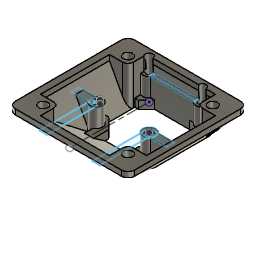
FanMod v4 (Autodesk Fusion 360 design; units mm, degrees)
Autodesk Fusion 360 part; units mm, degrees
note: some values were not read from the file. Chosen so that the rebuilt part matches the saved one: where a step ends; which bodies a step acts on; which sketch regions a step uses; which face or edge a step refers to.
sketch "2510Screws" plane through (0, 0, 0) normal (0, 0, 1) x (1, 0, 0)
  line L0 (12.5, -12.5) -> (-12.5, -12.5) construction
  line L1 (-12.5, -12.5) -> (-12.5, 12.5) construction
  line L2 (-12.5, 12.5) -> (12.5, 12.5) construction
  line L3 (12.5, 12.5) -> (12.5, -12.5) construction
  line L4 (12.5, -12.5) -> (-12.5, 12.5) construction
  line L5 (-12.5, -12.5) -> (12.5, 12.5) construction
  line L6 (10, -10) -> (-10, -10) construction
  line L7 (-10, -10) -> (-10, 10) construction
  line L8 (-10, 10) -> (10, 10) construction
  line L9 (10, 10) -> (10, -10) construction
  line L10 (10, -10) -> (-10, 10) construction
  line L11 (-10, -10) -> (10, 10) construction
  circle A0 centre (-10, 10) radius 1.4
  circle A1 centre (-10, -10) radius 1.4
  circle A2 centre (10, -10) radius 1.4
  circle A3 centre (10, 10) radius 1.4
  circle A4 centre (-10, 10) radius 2.4
  circle A5 centre (10, 10) radius 2.4
  circle A6 centre (-10, -10) radius 2.4
  circle A7 centre (10, -10) radius 2.4
  dimension "d1" = 25
  dimension "d2" = 25
  dimension "d3" = 20
  dimension "d4" = 20
  dimension "d5" = 2.8
  dimension "d6" = 2.8
  dimension "d7" = 2.8
  dimension "d8" = 2.8
  dimension "d9" = 4.8
  dimension "d10" = 4.8
  dimension "d11" = 4.8
  dimension "d12" = 4.8
  constraint horizontal L0
  constraint perpendicular L0 L1
  constraint parallel L0 L2
  constraint parallel L1 L3
  constraint coincident L4 origin
  constraint coincident L5 origin
  constraint horizontal L6
  constraint perpendicular L6 L7
  constraint parallel L6 L8
  constraint parallel L7 L9
  constraint coincident L10 origin
  constraint coincident L11 origin
  constraint coincident L7.end L8.start
  constraint coincident L6.end L7.start
  constraint coincident L6.start L9.end
  constraint coincident L8.end L9.start
  constraint concentric A0 A4
  constraint concentric A3 A5
  constraint concentric A1 A6
  constraint concentric A2 A7
  measures "d1" distance of L1.end L2.end
  measures "d2" distance of L0.end L1.end
  measures "d3" distance of L7.end L8.end
  measures "d4" distance of L6.end L7.end
  measures "d5" diameter of A0
  measures "d6" diameter of A1
  measures "d7" diameter of A2
  measures "d8" diameter of A3
  measures "d9" diameter of A4
  measures "d10" diameter of A5
  measures "d11" diameter of A6
  measures "d12" diameter of A7
sketch "Base" plane through (0, 0, 0) normal (0, 0, 1) x (1, 0, 0)
  line L0 (10, -12.5) -> (-10, -12.5)
  line L1 (-12.5, -10) -> (-12.5, 10)
  line L2 (-10, 12.5) -> (10, 12.5)
  line L3 (12.5, 10) -> (12.5, -10)
  line L4 (12.5, -12.5) -> (-12.5, 12.5) construction
  line L5 (-12.5, -12.5) -> (12.5, 12.5) construction
  arc A0 (-10, 12.5) -> (-12.5, 10) centre (-10, 10) ccw
  arc A1 (12.5, 10) -> (10, 12.5) centre (10, 10) ccw
  arc A2 (10, -12.5) -> (12.5, -10) centre (10, -10) ccw
  arc A3 (-12.5, -10) -> (-10, -12.5) centre (-10, -10) ccw
  line L6 (11, -11) -> (-11, -11)
  line L7 (-11, -11) -> (-11, 11)
  line L8 (-11, 11) -> (11, 11)
  line L9 (11, 11) -> (11, -11)
  line L10 (11, -11) -> (-11, 11) construction
  line L11 (-11, -11) -> (11, 11) construction
  dimension "d13" = 25
  dimension "d14" = 25
  dimension "d15" = 2.5
  dimension "d16" = 22
  dimension "d17" = 22
  constraint horizontal L0
  constraint perpendicular L0 L1
  constraint parallel L0 L2
  constraint parallel L1 L3
  constraint coincident L4 origin
  constraint coincident L5 origin
  constraint coincident L4.end L1
  constraint coincident L4.end L2
  constraint tangent L1 A0
  constraint tangent L2 A0
  constraint coincident L5.end L2
  constraint coincident L5.end L3
  constraint tangent L2 A1
  constraint tangent L3 A1
  constraint equal A0 A1
  constraint coincident L4.start L3
  constraint coincident L4.start L0
  constraint tangent L3 A2
  constraint tangent L0 A2
  constraint equal A0 A2
  constraint coincident L5.start L1
  constraint coincident L5.start L0
  constraint tangent L1 A3
  constraint tangent L0 A3
  constraint equal A0 A3
  constraint horizontal L6
  constraint perpendicular L6 L7
  constraint parallel L6 L8
  constraint parallel L7 L9
  constraint coincident L10 origin
  constraint coincident L11 origin
  measures "d13" distance of L4.end L5.end
  measures "d14" distance of L5.start L4.end
  measures "d15" radius of A0
  measures "d16" distance of L7.end L8.end
  measures "d17" distance of L6.end L7.end
ref_plane "WorkPlane1" through (0, 0, 13) normal (0, 0, 1) x (1, 0, 0)
sketch "Top" plane through (0, 0, 13) normal (0, 0, 1) x (1, 0, 0)
  line L0 (12.5, -12.5) -> (-12.5, -12.5) construction
  line L1 (-12.5, -12.5) -> (-12.5, 12.5) construction
  line L2 (-12.5, 12.5) -> (12.5, 12.5)
  line L3 (12.5, 12.5) -> (12.5, -12.5) construction
  line L4 (12.5, -12.5) -> (-12.5, 12.5) construction
  line L5 (-12.5, -12.5) -> (12.5, 12.5) construction
  line L6 (-12.5, 12.5) -> (-20.5, 12.5)
  line L7 (12.5, 12.5) -> (25.5, 12.5)
  line L8 (-18, 12.5) -> (22, 12.5)
  line L9 (24.5, 10) -> (24.5, -30)
  line L10 (22, -32.5) -> (-18, -32.5)
  line L11 (-20.5, -30) -> (-20.5, 10)
  line L12 (22, -30) -> (-18, -30)
  line L13 (-18, -30) -> (-18, 10)
  line L14 (-18, 10) -> (22, 10)
  line L15 (22, 10) -> (22, -30)
  line L16 (22, -30) -> (-18, 10) construction
  line L17 (-18, -30) -> (22, 10) construction
  arc A0 (-18, 12.5) -> (-20.5, 10) centre (-18, 10) ccw
  arc A1 (-20.5, -30) -> (-18, -32.5) centre (-18, -30) ccw
  arc A2 (22, -32.5) -> (24.5, -30) centre (22, -30) ccw
  arc A3 (24.5, 10) -> (22, 12.5) centre (22, 10) ccw
  line L18 (-18, 10) -> (-14, 10) construction
  line L19 (-14, 10) -> (-14, 6) construction
  line L20 (-14, 6) -> (-18, 6) construction
  line L21 (-18, 6) -> (-18, 10) construction
  line L22 (22, 10) -> (18, 10) construction
  line L23 (18, 10) -> (18, 6) construction
  line L24 (18, 6) -> (22, 6) construction
  line L25 (22, 6) -> (22, 10) construction
  line L26 (-18, -30) -> (-14, -30) construction
  line L27 (-14, -30) -> (-14, -26) construction
  line L28 (-14, -26) -> (-18, -26) construction
  line L29 (-18, -26) -> (-18, -30) construction
  line L30 (22, -30) -> (18, -30) construction
  line L31 (18, -30) -> (18, -26) construction
  line L32 (18, -26) -> (22, -26) construction
  line L33 (22, -26) -> (22, -30) construction
  circle A4 centre (-14, 6) radius 1.75
  circle A5 centre (-14, -26) radius 1.75
  circle A6 centre (18, -26) radius 1.75
  circle A7 centre (18, 6) radius 1.75
  line L34 (22, 10) -> (15, 10)
  line L35 (15, 10) -> (15, 5)
  line L36 (17, 3) -> (22, 3)
  line L37 (22, 3) -> (22, 10)
  line L38 (-18, 10) -> (-11, 10)
  line L39 (-11, 10) -> (-11, 5)
  line L40 (-13, 3) -> (-18, 3)
  line L41 (-18, 3) -> (-18, 10)
  line L42 (-18, -30) -> (-11, -30)
  line L43 (-11, -30) -> (-11, -25)
  line L44 (-13, -23) -> (-18, -23)
  line L45 (-18, -23) -> (-18, -30)
  line L46 (22, -30) -> (15, -30)
  line L47 (15, -30) -> (15, -25)
  line L48 (17, -23) -> (22, -23)
  line L49 (22, -23) -> (22, -30)
  arc A8 (-13, 3) -> (-11, 5) centre (-13, 5) ccw
  arc A9 (-11, -25) -> (-13, -23) centre (-13, -25) ccw
  arc A10 (17, -23) -> (15, -25) centre (17, -25) ccw
  arc A11 (15, 5) -> (17, 3) centre (17, 5) ccw
  point P0 (24.5, 12.5)
  point P1 (-20.5, -32.5)
  point P2 (2, -10)
  dimension "d19" = 25
  dimension "d20" = 25
  dimension "d21" = 8
  dimension "d22" = 13
  dimension "d23" = 45
  dimension "d24" = 45
  dimension "d25" = 40
  dimension "d26" = 40
  dimension "d27" = 2.5
  dimension "d28" = 4
  dimension "d29" = 4
  dimension "d30" = 4
  dimension "d31" = 4
  dimension "d32" = 4
  dimension "d33" = 4
  dimension "d34" = 4
  dimension "d35" = 4
  dimension "d36" = 3.5
  dimension "d37" = 3.5
  dimension "d38" = 3.5
  dimension "d39" = 3.5
  dimension "d40" = 7
  dimension "d41" = 7
  dimension "d42" = 7
  dimension "d43" = 7
  dimension "d44" = 7
  dimension "d45" = 7
  dimension "d46" = 7
  dimension "d47" = 7
  dimension "d48" = 2
  constraint horizontal L0
  constraint perpendicular L0 L1
  constraint parallel L0 L2
  constraint parallel L1 L3
  constraint coincident L4 origin
  constraint coincident L5 origin
  constraint perpendicular L1 L6
  constraint perpendicular L3 L7
  constraint horizontal L8
  constraint vertical L9
  constraint horizontal L10
  constraint vertical L11
  constraint horizontal L12
  constraint perpendicular L12 L13
  constraint parallel L12 L14
  constraint parallel L13 L15
  constraint coincident L16 P2
  constraint coincident L17 P2
  constraint coincident L6.end L11
  constraint coincident L6.end L8
  constraint tangent L11 A0
  constraint tangent L8 A0
  constraint coincident P1 L11
  constraint coincident P1 L10
  constraint tangent L11 A1
  constraint tangent L10 A1
  constraint equal A0 A1
  constraint tangent L10 A2
  constraint tangent L9 A2
  constraint equal A0 A2
  constraint coincident P0 L9
  constraint coincident P0 L8
  constraint tangent L9 A3
  constraint tangent L8 A3
  constraint equal A0 A3
  constraint horizontal L18
  constraint vertical L19
  constraint horizontal L20
  constraint vertical L21
  constraint coincident L13.end L14.start
  constraint horizontal L22
  constraint vertical L23
  constraint horizontal L24
  constraint vertical L25
  constraint coincident L14.end L15.start
  constraint horizontal L26
  constraint vertical L27
  constraint horizontal L28
  constraint vertical L29
  constraint coincident L12.end L13.start
  constraint horizontal L30
  constraint vertical L31
  constraint horizontal L32
  constraint vertical L33
  constraint coincident L12.start L15.end
  constraint coincident L19.end L20.start
  constraint coincident L27.end L28.start
  constraint coincident L31.end L32.start
  constraint coincident L23.end L24.start
  constraint horizontal L34
  constraint vertical L35
  constraint horizontal L36
  constraint vertical L37
  constraint horizontal L38
  constraint vertical L39
  constraint horizontal L40
  constraint vertical L41
  constraint horizontal L42
  constraint vertical L43
  constraint horizontal L44
  constraint vertical L45
  constraint horizontal L46
  constraint vertical L47
  constraint horizontal L48
  constraint vertical L49
  constraint tangent L39 A8
  constraint tangent L40 A8
  constraint tangent L43 A9
  constraint tangent L44 A9
  constraint equal A8 A9
  constraint tangent L47 A10
  constraint tangent L48 A10
  constraint equal A8 A10
  constraint tangent L35 A11
  constraint tangent L36 A11
  constraint equal A8 A11
  measures "d19" distance of L1.end L2.end
  measures "d20" distance of L0.end L1.end
  measures "d21" distance of L1.end L6.end
  measures "d22" distance of L2.end L7.end
  measures "d23" distance of L6.end P0
  measures "d24" distance of L6.end P1
  measures "d25" distance of L13.end L14.end
  measures "d26" distance of L12.end L13.end
  measures "d27" radius of A0
  measures "d28" distance of L13.end L18.end
  measures "d29" distance of L13.end L20.end
  measures "d30" distance of L14.end L22.end
  measures "d31" distance of L14.end L24.end
  measures "d32" distance of L12.end L26.end
  measures "d33" distance of L12.end L28.end
  measures "d34" distance of L12.start L30.end
  measures "d35" distance of L12.start L32.end
  measures "d36" diameter of A4
  measures "d37" diameter of A5
  measures "d38" diameter of A6
  measures "d39" diameter of A7
  measures "d40" distance of L14.end L34.end
  measures "d41" distance of L14.end L36.end
  measures "d42" distance of L13.end L38.end
  measures "d43" distance of L13.end L40.end
  measures "d44" distance of L12.end L42.end
  measures "d45" distance of L12.end L44.end
  measures "d46" distance of L12.start L46.end
  measures "d47" distance of L12.start L48.end
  measures "d48" radius of A8
loft "Loft3" add profiles "Base", "Top" section 1 section 2 contours L2 L6 L7 L8 L9 L10 L11 A0 A1 A2 A3 | L12 L15 L46 L47 L48 L49 A10 | L12 L13 L14 L15 L35 L36 L39 L40 L43 L44 L47 L48 A8 A9 A10 A11 | L12 L13 L42 L43 L44 L45 A9 | L14 L15 L34 L35 L36 L37 A11 | L13 L14 L38 L39 L40 L41 A8 | A4 | A5 | A6 | A7 makes body 1
loft "Loft4" cut profiles "Top", "Base" section 1 contours L12 L15 L46 L47 L48 L49 A10 | L12 L13 L14 L15 L35 L36 L39 L40 L43 L44 L47 L48 A8 A9 A10 A11 | L12 L13 L42 L43 L44 L45 A9 | L14 L15 L34 L35 L36 L37 A11 | L13 L14 L38 L39 L40 L41 A8 section 2 contours L6 L7 L8 L9 bodies 1
extrude "Extrude4" add sketch "Top" along normal up to far side of body 1 contours L12 L15 L46 L47 L48 L49 A10 | L12 L13 L42 L43 L44 L45 A9 | L14 L15 L34 L35 L36 L37 A11 | L13 L14 L38 L39 L40 L41 A8 bodies 1
extrude "Extrude5" cut sketch "Top" against normal blind 12 contours A4 | A5 | A6 | A7 bodies 1
extrude "Extrude6" add sketch "Top" along normal blind 2 contours L2 L6 L7 L8 L9 L10 L11 A0 A1 A2 A3 | L12 L15 L46 L47 L48 L49 A10 | L12 L13 L42 L43 L44 L45 A9 | L14 L15 L34 L35 L36 L37 A11 | L13 L14 L38 L39 L40 L41 A8 bodies 1
extrude "Extrude7" add sketch "2510Screws" along normal blind 10 bodies 1
extrude "Extrude8" cut sketch "2510Screws" along normal blind 22 contours A0 | A3 bodies 1
extrude "Extrude9" cut sketch "2510Screws" along normal blind 10 contours A1 | A2 bodies 1
sketch "ReinforcementBottom" plane through (0, 0, 0) normal (0, 0, 1) x (1, 0, 0)
  line L0 (-11, -11) -> (-5.6, -11)
  line L1 (-5.6, -11) -> (-5.6, -9.8071)
  line L2 (-9.8071, -5.6) -> (-11, -5.6)
  line L3 (-11, -5.6) -> (-11, -11)
  line L4 (11, -11) -> (5.6, -11)
  line L5 (5.6, -11) -> (5.6, -9.8071)
  line L6 (9.6, -5.6) -> (11, -5.6)
  line L7 (11, -5.6) -> (11, -11)
  line L8 (-11, 11) -> (-5.6, 11)
  line L9 (-5.6, 11) -> (-5.6, 9.6)
  line L10 (-9.6, 5.6) -> (-11, 5.6)
  line L11 (-11, 5.6) -> (-11, 11)
  line L12 (11, 11) -> (5.6, 11)
  line L13 (5.6, 11) -> (5.6, 9.6)
  line L14 (9.6, 5.6) -> (11, 5.6)
  line L15 (11, 5.6) -> (11, 11)
  line L16 (-5.6, 9.6) -> (-9.6, 5.6)
  line L17 (-5.7464, -9.4536) -> (-9.4536, -5.7464)
  line L18 (5.7464, -9.4536) -> (9.6, -5.6)
  line L19 (5.6, 9.6) -> (9.6, 5.6)
  arc A0 (-9.4536, -5.7464) -> (-9.8071, -5.6) centre (-9.8071, -6.1) ccw
  arc A1 (-5.6, -9.8071) -> (-5.7464, -9.4536) centre (-6.1, -9.8071) ccw
  arc A2 (5.7464, -9.4536) -> (5.6, -9.8071) centre (6.1, -9.8071) ccw
  point P0 (-5.6, -5.6)
  point P1 (5.6, -5.6)
  point P2 (-5.6, 5.6)
  point P3 (5.6, 5.6)
  point P4 (-5.6, -9.6)
  point P5 (-9.6, -5.6)
  point P6 (5.6, -9.6)
  dimension "d64" = 5.4
  dimension "d65" = 5.4
  dimension "d66" = 5.4
  dimension "d67" = 5.4
  dimension "d68" = 5.4
  dimension "d69" = 5.4
  dimension "d70" = 5.4
  dimension "d71" = 5.4
  dimension "d72" = 4
  dimension "d73" = 4
  dimension "d74" = 4
  dimension "d75" = 4
  dimension "d76" = 4
  dimension "d77" = 4
  dimension "d78" = 4
  dimension "d79" = 4
  dimension "d80" = 0.5
  constraint horizontal L0
  constraint vertical L1
  constraint horizontal L2
  constraint vertical L3
  constraint horizontal L4
  constraint vertical L5
  constraint horizontal L6
  constraint vertical L7
  constraint horizontal L8
  constraint vertical L9
  constraint horizontal L10
  constraint vertical L11
  constraint horizontal L12
  constraint vertical L13
  constraint horizontal L14
  constraint vertical L15
  constraint coincident P2 L9
  constraint coincident P2 L10
  constraint coincident P0 L1
  constraint coincident P0 L2
  constraint coincident P1 L5
  constraint coincident P1 L6
  constraint coincident P3 L13
  constraint coincident P3 L14
  constraint coincident P5 L17
  constraint coincident L2 P5
  constraint tangent L17 A0
  constraint tangent L2 A0
  constraint coincident P4 L17
  constraint coincident L1 P4
  constraint tangent L17 A1
  constraint tangent L1 A1
  constraint equal A0 A1
  constraint coincident P6 L18
  constraint coincident L5 P6
  constraint tangent L18 A2
  constraint tangent L5 A2
  constraint equal A0 A2
  measures "d64" distance of L0.start L0.end
  measures "d65" distance of L0.start L2.end
  measures "d66" distance of L4.start L4.end
  measures "d67" distance of L4.start L6.end
  measures "d68" distance of L8.start L8.end
  measures "d69" distance of L8.start L10.end
  measures "d70" distance of L12.start L12.end
  measures "d71" distance of L12.start L14.end
  measures "d72" distance of P2 L9.end
  measures "d73" distance of P2 L10.start
  measures "d74" distance of P0 P4
  measures "d75" distance of P0 P5
  measures "d76" distance of P1 P6
  measures "d77" distance of P1 L6.start
  measures "d78" distance of P3 L13.end
  measures "d79" distance of P3 L14.start
  measures "d80" radius of A0
extrude "Extrude10" add sketch "ReinforcementBottom" along normal blind 3 separate body makes body 2 at (-8.7333, 8.7333, 0) makes body 3 at (-8.7333, -8.7333, 0) makes body 4 at (8.7333, 8.7333, 0) makes body 5 at (8.7821, -8.6845, 0)
extrude "Extrude11" cut sketch "2510Screws" along normal blind 10 contours A0 | A1 | A2 | A3 bodies 2 3 4 5 makes body 9 at (10.9821, -10.9978, 1) makes body 8 at (10.9888, 10.9911, 2) makes body 7 at (-8.07, -8.07, 3) makes body 6 at (-10.9888, 10.9911, 1)
extrude "Extrude12" add 1 faces at (7.8801, -11, 2) along direction (0, -1, 0) up to surface end surface at (8.9798, -17.8527, 4.6887) on bodies 1 5 bodies 1 2 3 4 6 7 8 9 5
extrude "Extrude13" add 1 faces at (-6.7401, -11, 1) along direction (0, -1, 0) up to surface end surface at (6.1034, -27.5481, 11.3224) on bodies 1 7 bodies 1 2 3 4 6 8 9 7
extrude "Extrude14" add 1 faces at (-11, -6.3394, 1) along direction (-1, 0, 0) up to surface end surface at (-14.399, -3.1368, 6.3124) on bodies 1 bodies 1
extrude "Extrude15" add 1 faces at (11, -6.3394, 1) along direction (1, 0, 0) up to surface end surface at (21.1667, -9.6242, 12.0152) on bodies 1 bodies 1
extrude "Extrude16" add 1 faces at (11, 7.8801, 2) along direction (1, 0, 0) up to surface end surface at (21.1667, -9.6242, 12.0152) on bodies 1 4 bodies 1 2 3 6 8 9 4
sketch "ReinforcementTop" plane through (0, 0, 10) normal (0, 0, 1) x (-1, 0, 0)
  circle A0 centre (10, 10) radius 1.4
  circle A1 centre (10, 10) radius 2.4
  line L0 (10, 8.6) -> (18, 8.6)
  line L1 (18, 8.6) -> (18, 11.4)
  line L2 (18, 11.4) -> (10, 11.4)
  line L3 (10, 11.4) -> (10, 8.6)
  line L4 (8.6, 10) -> (11.4, 10)
  line L5 (11.4, 10) -> (11.4, 30)
  line L6 (11.4, 30) -> (8.6, 30)
  line L7 (8.6, 30) -> (8.6, 10)
  line L8 (8.5, -10) -> (-8.5, -10)
  line L9 (-8.5, -10) -> (-8.5, -8.6)
  line L10 (-8.5, -8.6) -> (8.5, -8.6)
  line L11 (8.5, -8.6) -> (8.5, -10)
  line L12 (0, 0) -> (0, 30)
  line L13 (-8.6, 30) -> (-8.6, 10)
  line L14 (-8.6, 10) -> (-11.4, 10)
  line L15 (-10, 11.4) -> (-10, 8.6)
  line L16 (-10, 8.6) -> (-18, 8.6)
  line L17 (-18, 11.4) -> (-10, 11.4)
  line L18 (-11.4, 10) -> (-11.4, 30)
  line L19 (-11.4, 30) -> (-8.6, 30)
  line L20 (-18, 8.6) -> (-18, 11.4)
  circle A2 centre (-10, 10) radius 2.4
  dimension "d96" = 2.8
  dimension "d97" = 20
  dimension "d98" = 17
  dimension "d99" = 1.4
  dimension "d100" = 4.8
  constraint horizontal L0
  constraint vertical L1
  constraint horizontal L2
  constraint vertical L3
  constraint coincident A0 L0.start
  constraint horizontal L4
  constraint vertical L5
  constraint horizontal L6
  constraint vertical L7
  constraint coincident A0 L4.start
  constraint horizontal L8
  constraint vertical L9
  constraint horizontal L10
  constraint vertical L11
  constraint coincident L12.start origin
  constraint vertical L12
  constraint symmetric L0.start L12 L15.end
  constraint symmetric L0.end L12 L16.end
  constraint symmetric L1.end L12 L17.start
  constraint symmetric L2.end L12 L15.start
  constraint symmetric L4.start L12 L13.end
  constraint symmetric L4.end L12 L14.end
  constraint symmetric L5.end L12 L18.end
  constraint symmetric L6.end L12 L13.start
  constraint midpoint L15 A2.centre
  measures "d96" distance of L4.start L4.end
  measures "d97" distance of L4.start L6.end
  measures "d98" distance of L8.start L8.end
  measures "d99" distance of L8.start L10.end
  measures "d100" diameter of A2
extrude "Extrude17" add sketch "ReinforcementTop" along normal up to far side of body 1 contours A1 L0 L1 L2 | L16 L17 L20 A2 bodies 1
extrude "Extrude18" add sketch "ReinforcementTop" against normal blind 10 contours L8 L9 L10 L11 bodies 1 2
equation "d73 = d72"
equation "d75 = d74"
equation "d77 = d76"
equation "d79 = d78"
